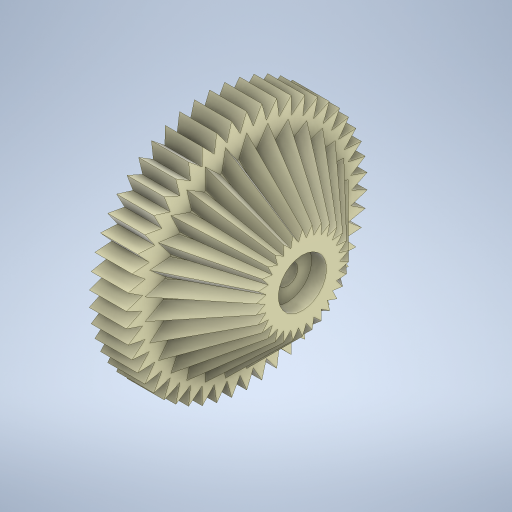
# Autodesk Inventor part: Bevel Gear
Saved by Autodesk Inventor 2023 (Build 270158030, 158C)
## iProperties
Created: 2022-09-21
Part Number: Bevel Gear
Material: Polypropylene
Document SubType Name: Modeling
Designer: caden
Density: 0.899 g/cm^3
Appearance: Smooth - Ash
Author: caden
Autodesk Inventor part; units mm, degrees
ref_plane "YZ Plane" through (0, 0, 0) normal (1, 0, 0) x (0, 1, 0)
ref_plane "XZ Plane" through (0, 0, 0) normal (0, 1, 0) x (-1, 0, 0)
ref_plane "XY Plane" through (0, 0, 0) normal (0, 0, 1) x (1, 0, 0)
sketch "Sketch1" plane through (0, 0, 0) normal (0, 0, 1) x (1, 0, 0)
  line L0 (20, 45) -> (50, 15)
  line L1 (50, 15) -> (50, 0)
  line L2 (50, 0) -> (0, 0)
  line L3 (0, 0) -> (0, 55)
  line L4 (0, 0) -> (65.4619, 0)
  line L5 (20, 45) -> (20, 55)
  line L6 (20, 55) -> (0, 55)
  dimension "d1" = 45
  dimension "d2" = 30
  dimension "d50" = 20
  dimension "d51" = 10
  dimension "d52" = 50
  constraints: 14 end point, 2 horizontal, 2 perpendicular, 1 point on line, 1 vertical
  measures "d1" angle of L4 L0
  measures "d2" diameter of L0.end L4
  measures "d50" distance of L5.end L3.end
  measures "d51" distance of L0.start L5.end
  measures "d52" distance between parallel lines of L3 L1
revolve "Main Body" add sketch "Sketch1" angle 360 about axis through (0, 0, 0) along (1, 0, 0)
sketch "Sketch16" plane through (20, 0, 0) normal (1, 0, 0) x (0, 0, -1)
  circle A0 centre (0, 0) radius 45 projected
  line L0 (-4.2245, 44.8013) -> (0, 55)
  line L1 (0, 55) -> (4.2245, 44.8013)
  line L2 (0, 0) -> (0, 68.3792)
  arc A1 (13.6554, 42.8781) -> (-4.2245, 44.8013) centre (0, 0) ccw
  point P0 (0, 45)
  dimension "d53" = 45
  dimension "d54" = 10
  constraints: 6 end point, 6 point on circle, 2 point on line, 1 centre point, 1 concentric, 1 symmetric about line, 1 vertical
  measures "d53" angle of L1 L0
  measures "d54" distance of L0.end point (0, 45)
sketch "Sketch17" plane through (50, 0, 0) normal (1, 0, 0) x (0, 0, -1)
  circle A0 centre (0, 0) radius 15 projected
  line L0 (0, 0) -> (0, 17.3651)
  line L1 (0, 25) -> (-4.4177, 14.3347)
  line L2 (0, 25) -> (4.4177, 14.3347)
  arc A1 (4.4177, 14.3347) -> (-4.4177, 14.3347) centre (0, 0) ccw
  point P0 (0, 15)
  dimension "d55" = 45
  dimension "d56" = 10
  constraints: 6 end point, 5 point on circle, 1 centre point, 1 concentric, 1 point on line, 1 symmetric about line, 1 vertical
  measures "d55" angle of L2 L1
  measures "d56" distance of L1.start point (0, 15)
loft "Loft3" add profiles "Sketch17", "Sketch16" contours A0 L1 L2 / L0 L2 A0 | A0 L2 L1
pattern_circular "Circular Pattern4" count 30 over 360 about axis through (35, 0, 0) along (1, 0, 0) of "Loft3"
sketch "Sketch18" plane through (50, 19.9403, -2.0958) normal (1, 0, 0) x (0, 0.3827, -0.9239)
  circle A0 centre (-9.5671, -17.6204) radius 13
  dimension "d64" = 26
  constraints: 1 centre point, 1 coincident
  measures "d64" diameter of A0
extrude "Extrusion7" cut sketch "Sketch18" against normal blind 8
sketch "Sketch19" plane through (42, 0, 0) normal (1, 0, 0) x (0, 0, -1)
  circle A0 centre (0, 0) radius 5.5
  dimension "d67" = 11
  constraints: 1 centre point, 1 coincident
  measures "d67" diameter of A0
extrude "Extrusion8" cut sketch "Sketch19" against normal through all
sketch "Sketch20" plane through (0, 0, 0) normal (-1, 0, 0) x (0, 0, 1)
  circle A0 centre (0, 0) radius 5.5 projected
  circle A1 centre (0, 0) radius 13
  dimension "d70" = 26
  constraints: 1 centre point, 1 coincident
  measures "d70" diameter of A1
extrude "Extrusion9" cut sketch "Sketch20" against normal blind 8
sketch "Sketch21" plane through (20, 0, 0) normal (1, 0, 0) x (0, 0, -1)
  circle A0 centre (0, 0) radius 55 projected
  line L0 (-4.2089, 54.8387) -> (0, 65)
  line L1 (0, 65) -> (4.2089, 54.8387)
  line L2 (0, 0) -> (0, 84.4884)
  arc A1 (4.2089, 54.8387) -> (-4.2089, 54.8387) centre (0, 0) ccw
  point P0 (0, 55)
  dimension "d73" = 10
  dimension "d74" = 45
  constraints: 6 end point, 5 point on circle, 1 centre point, 1 concentric, 1 point on line, 1 symmetric about line, 1 vertical
  measures "d73" distance of L0.end point (0, 55)
  measures "d74" angle of L1 L0
extrude "Extrusion10" add sketch "Sketch21" against normal up to surface (20 mm away) contours A0 L2 L1 | L0 L2 A0
pattern_circular "Circular Pattern5" count 50 over 360 about axis through (10, 0, 0) along (1, 0, 0) of "Extrusion10"
body "Solid1"
